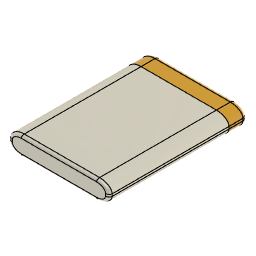
combined_hardware_electronics_OSSG_v1 (Autodesk Fusion 360 archive; units mm, degrees)
design "ear_battery_to_scale"
Autodesk Fusion 360 part; units mm, degrees
sketch "Sketch3" plane through (0, 0, 0) normal (0, 0, 1) x (1, 0, 0)
  line L0 (14, -23) -> (-14, -23)
  line L1 (-14, -23) -> (-14, 23)
  line L2 (-14, 23) -> (14, 23)
  line L3 (14, 23) -> (14, -23)
  line L4 (14, -23) -> (-14, 23) construction
  line L5 (-14, -23) -> (14, 23) construction
  line L6 (-14, 17.0852) -> (14, 17.0852)
  dimension "d7" = 28
  dimension "d8" = 46
  constraint horizontal L0
  constraint perpendicular L0 L1
  constraint parallel L0 L2
  constraint parallel L1 L3
  constraint coincident L4 origin
  constraint coincident L5 origin
  constraint coincident L1 L6.start
  constraint coincident L3 L6.end
  constraint perpendicular L3 L6
  measures "d7" distance of L1.end L2.end
  measures "d8" distance of L0.end L1.end
extrude "Extrude2" add sketch "Sketch3" along normal blind 8 contours L0 L1 L3 L6 makes body 1
extrude "Extrude3" add sketch "Sketch3" along normal blind 8 separate body contours L1 L2 L3 L6 makes body 2
fillet "Fillet2" radius 3.5 8 edges at (-14, -2.9574, 8) (-14, -2.9574, 0) (14, -2.9574, 8) (14, -2.9574, 0) (-14, 20.0426, 0) (-14, 20.0426, 8) (14, 20.0426, 8) (14, 20.0426, 0) on bodies 1 2
sketch "Sketch4" plane through (0, 23, 0) normal (0, 1, 0) x (-1, 0, 0)
  arc A0 (-14, 3.5) -> (-10.5, 0) centre (-10.5, 3.5) ccw
  line L0 (-10.5, 0) -> (10.5, 0)
  arc A1 (10.5, 0) -> (14, 3.5) centre (10.5, 3.5) ccw
  line L1 (14, 3.5) -> (14, 4.5)
  arc A2 (14, 4.5) -> (10.5, 8) centre (10.5, 4.5) ccw
  line L2 (10.5, 8) -> (-10.5, 8)
  arc A3 (-10.5, 8) -> (-14, 4.5) centre (-10.5, 4.5) ccw
  line L3 (-14, 4.5) -> (-14, 3.5)
  circle A4 centre (-12, 3) radius 0.5
  circle A5 centre (-12, 4.5) radius 0.5
  dimension "d15" = 1
  dimension "d16" = 1
  measures "d15" diameter of A4
  measures "d16" diameter of A5
fillet "Fillet3" radius 1.25 1 faces at (3.5, 23, 5.3333) on bodies 2
fillet "Fillet4" radius 1 1 faces at (-3.5, -23, 5.3333) on bodies 1
extrude "Extrude4" add sketch "Sketch4" along normal blind 0.2 separate body contours A4 | A5 makes body 3 at (11.756, 23, 4.6134) makes body 4 at (12.0371, 23, 3.1625)
scale "Scale1" factors (0.8, 0.66667, 0.5) about (10.5, 23, 6.75) bodies 1 2 3 4
named bodies: "battery", "overcharging electronics", "ground wire", "power wire"
